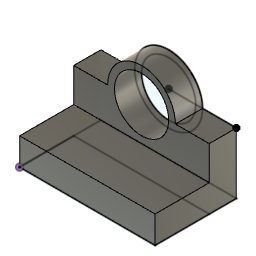
Exercise 3 v1 (Autodesk Fusion 360 design; units mm, degrees)
Autodesk Fusion 360 part; units mm, degrees
note: some values were not read from the file. Set by a fixed rule: which sketch regions a step uses.
sketch "Sketch1" plane through (0, 0, 0) normal (0, 0, 1) x (1, 0, 0)
  line L0 (0, 0) -> (100, 0)
  line L1 (100, 0) -> (100, 60)
  line L2 (100, 60) -> (0, 60)
  line L3 (0, 60) -> (0, 0)
  line L4 (0, 0) -> (0, 40)
  line L5 (0, 40) -> (100, 40)
  dimension "d1" = 100
  dimension "d2" = 60
  dimension "d3" = 40
  constraint horizontal L0
  constraint vertical L1
  constraint horizontal L2
  constraint vertical L3
  constraint coincident L0.start L3.end
  constraint perpendicular L0 L4
  constraint coincident L1 L5.end
  constraint perpendicular L1 L5
  measures "d1" distance of L0.start L0.end
  measures "d2" distance of L0.start L2.end
  measures "d3" distance of L0.start L4.end
extrude "Extrude1" add sketch "Sketch1" along normal blind 20 contours L0 L1 L3 L4 L5
extrude "Extrude2" add sketch "Sketch1" along normal blind 45 contours L1 L2 L3 L5
sketch "Sketch2" plane through (0, 60, 0) normal (0, 1, 0) x (-1, 0, 0)
  line L0 (-100, 0) -> (0, 0)
  line L1 (0, 0) -> (0, 45)
  line L2 (0, 45) -> (-100, 45)
  line L3 (-100, 45) -> (-100, 0)
  line L4 (-100, 45) -> (-50, 45)
  circle A0 centre (-50, 45) radius 20
  circle A1 centre (-50, 45) radius 25
  dimension "d8" = 50
  dimension "d9" = 40
  dimension "d10" = 50
  constraint coincident L2.end L3.start
  constraint perpendicular L3 L4
  constraint coincident L4.end A0.centre
  constraint concentric A0 A1
  measures "d8" distance of L2.end L4.end
  measures "d9" diameter of A0
  measures "d10" diameter of A1
extrude "Extrude3" add sketch "Sketch2" against normal blind 20 contours L2 L4 A0 A1 picked at (-37.3043, 64.5056)
extrude "Extrude4" cut sketch "Sketch2" against normal blind 20 contours L2 L4 A0 picked at (-36.7411, 44.0064)
